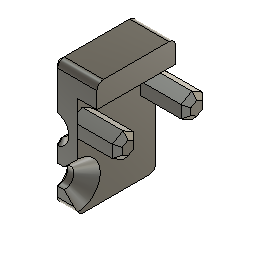
Omron v2_1 Mount (Autodesk Fusion 360 design; units mm, degrees)
Autodesk Fusion 360 part; units mm, degrees
sketch "Sketch1" plane through (0, 0, 0) normal (0, 1, 0) x (1, 0, 0)
  line L0 (0, 0) -> (0, -19.1)
  line L1 (0, -19.1) -> (6.5, -19.1)
  line L2 (6.5, -19.1) -> (6.5, -15.6)
  line L3 (6.5, -15.6) -> (3.5, -15.6)
  line L4 (3.5, -15.6) -> (3.5, 0)
  line L5 (3.5, 0) -> (0, 0)
  dimension "d1" = 3.5
  dimension "d2" = 15.6
  dimension "d3" = 3
  constraint coincident L0.start L5.end
  constraint vertical L0
  constraint perpendicular L0 L1
  constraint perpendicular L1 L2
  constraint perpendicular L2 L3
  constraint perpendicular L3 L4
  constraint perpendicular L0 L5
  constraint equal L2 L5
  measures "d1" distance of L0.start L4.end
  measures "d2" distance of L3.end L4.end
  measures "d3" distance of L2.end L3.end
extrude "Extrude1" add sketch "Sketch1" along normal blind 17 makes body 1
ref_plane "WorkPlane3" through (3.25, 8.5, 9.55) normal (0, -1, 0) x (-1, 0, 0)
sketch "Sketch2" plane through (3.5, 0, 0) normal (1, 0, 0) x (0, 1, 0)
  line L0 (2.5, 0) -> (14.5, 0)
  line L1 (14.5, 15.6) -> (2.5, 15.6)
  circle A0 centre (3.25, 12.15) radius 1.9 construction
  circle A1 centre (13.75, 12.15) radius 1.9 construction
  line L2 (4.8954, 13.1) -> (3.25, 14.05)
  line L3 (3.25, 14.05) -> (1.6046, 13.1)
  line L4 (1.6046, 13.1) -> (1.6046, 11.2)
  line L5 (1.6046, 11.2) -> (3.25, 10.25)
  line L6 (3.25, 10.25) -> (4.8954, 11.2)
  line L7 (4.8954, 11.2) -> (4.8954, 13.1)
  line L8 (15.3954, 13.1) -> (13.75, 14.05)
  line L9 (13.75, 14.05) -> (12.1046, 13.1)
  line L10 (12.1046, 13.1) -> (12.1046, 11.2)
  line L11 (12.1046, 11.2) -> (13.75, 10.25)
  line L12 (13.75, 10.25) -> (15.3954, 11.2)
  line L13 (15.3954, 11.2) -> (15.3954, 13.1)
  line L14 (8.5, -1.91) -> (8.5, 21.01)
  line L15 (2.5, 15.6) -> (2.5, 0)
  line L16 (14.5, 0) -> (14.5, 15.6)
  point P0 (3.25, 12.15)
  point P1 (13.75, 12.15)
  dimension "d6" = 3.8
  dimension "d7" = 3.8
  dimension "d8" = 3.45
  dimension "d9" = 3.45
  dimension "d11" = 10.5
  dimension "d53" = 5.25
  constraint coincident P0 A0.centre
  constraint coincident A0 L2.start
  constraint coincident P1 A1.centre
  constraint coincident A1 L8.start
  constraint vertical L13
  constraint vertical L4
  measures "d6" diameter of A0
  measures "d7" diameter of A1
  measures "d8" distance of L1 P1
  measures "d9" distance of L1 P0
  measures "d11" distance of P0 P1
  measures "d53" distance of P0 L14
ref_plane "WorkPlane1" through (3.25, 14.5, 9.55) normal (0, 1, 0) x (0, 0, 1)
split "Split1" by plane through (3.25, 14.5, 9.55) normal (0, 1, 0) bodies 1 makes body 2 at (1.1667, 17, 11.5667)
delete_body "RemoveBody1" bodies 2
ref_plane "WorkPlane2" through (3.25, 2.5, 9.55) normal (0, -1, 0) x (-1, 0, 0)
split "Split2" by plane through (3.25, 2.5, 9.55) normal (0, -1, 0) bodies 1 makes body 3 at (1.1667, 0, 11.5667)
delete_body "RemoveBody2" bodies 3
extrude "Extrude2" add sketch "Sketch2" along normal blind 7 contours L2 L3 L5 L6 L7 L15 | L3 L4 L5 L15 | L8 L12 L13 L16 | L8 L9 L10 L11 L12 L16 bodies 1
hole "Hole6" at (0, 2.5, 10) direction (0, 1, 0) diameter 2.95 depth 12 tip angle 118 bodies 1
chamfer "Chamfer1" distance 0.75 angle 45 2 edges at (1.475, 2.5, 10) (1.475, 14.5, 10) on bodies 1
thread "Thread3" [suppressed]
fillet "Fillet2" radius 1 4 edges at (3.25, 2.5, 19.1) (1.75, 2.5, 0) (3.25, 14.5, 19.1) (1.75, 14.5, 0) on bodies 1
sketch "Sketch4" plane through (0, 0, 19.1) normal (0, 0, 1) x (-1, 0, 0)
  line L0 (-6.5, -13.5) -> (0, -13.5)
  line L1 (0, -13.5) -> (0, -3.5)
  line L2 (0, -3.5) -> (-6.5, -3.5)
  line L3 (-6.5, -3.5) -> (-6.5, -13.5)
  line L4 (0, -2.5) -> (-6.5, -2.5)
  line L5 (-3.5, -1.6046) -> (-10.5, -1.6046)
  line L6 (-6.5, -14.5) -> (0, -14.5)
  line L7 (-3.5, -15.3954) -> (-10.5, -15.3954)
  line L8 (-3.5, -15.3954) -> (-3.5, -14.5)
  line L9 (-3.5, -14.5) -> (-3.5, -15.3954)
  line L10 (-3.5, -14.5) -> (-4.3954, -15.3954)
  line L11 (-4.3954, -15.3954) -> (-3.5, -15.3954)
  line L12 (-3.5, -1.6046) -> (-3.5, -2.5)
  line L13 (-3.5, -2.5) -> (-4.3954, -1.6046)
  line L14 (-4.3954, -1.6046) -> (-3.5, -1.6046)
  dimension "d65" = 45
  dimension "d66" = 45
  constraint coincident L8.end L9.start
  constraint coincident L7.start L8.start
  constraint coincident L7 L10.end
  constraint coincident L5.start L12.start
  constraint coincident L4 L12.end
  constraint perpendicular L4 L12
  constraint coincident L5 L13.end
  measures "d65" angle of L9 L10
  measures "d66" angle of L12 L13
extrude "Extrude5" cut sketch "Sketch4" against normal up to surface (19.1 mm away) contours L5 L12 L13 L14 | L7 L8 L9 L10 L11 bodies 1
hole "Hole7" at (3.5, 2.5, 4) direction (-1, 0, 0) diameter 3 end through all bodies 1
chamfer "Chamfer3" distance 0.5 angle 45 18 edges at (0, 14.5, 15.1625) (0, 14.2071, 18.8071) (0, 8.5, 19.1) (0, 2.7929, 18.8071) (0, 2.5, 15.1625) (0, 2.875, 11.85) (0, 14.125, 11.85) (0, 8.5, 11.475) (0, 8.5, 8.525) (0, 14.125, 8.15) (0, 2.875, 8.15) (0, 2.5, 6.6375) (0, 2.5, 1.75) (0, 2.7929, 0.2929) (0, 8.5, 0) (0, 14.2071, 0.2929) (0, 14.5, 4.3875) (0, 4, 4) on bodies 1
chamfer "Chamfer4" distance 0.75 angle 45 12 edges at (10.5, 12.9273, 13.575) (10.5, 12.1046, 12.15) (10.5, 12.9273, 10.725) (10.5, 14.5727, 10.725) (10.5, 15.3954, 12.15) (10.5, 14.5727, 13.575) (10.5, 4.0727, 13.575) (10.5, 2.4273, 13.575) (10.5, 1.6046, 12.15) (10.5, 2.4273, 10.725) (10.5, 4.0727, 10.725) (10.5, 4.8954, 12.15) on bodies 1
chamfer "Chamfer5" distance 2 angle 45 1 edges at (3.5, 4, 4) on bodies 1
